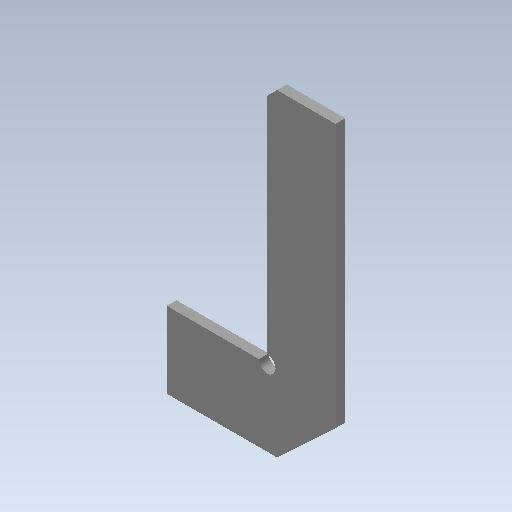
# Autodesk Inventor part: ADSK-MH-10038
Saved by Autodesk Inventor 2020.2 (Build 242310000, 310)
## iProperties
Created: 2008-03-27
Part Number: ADSK-MH-10038
Document SubType Name: Modeling
Designer: R.O'mahony
Density: 7.86 g/cm^3
Mass: 284.494 g
Surface Area: 169.314 cm^2
Volume: 36.1952 cm^3
Material: Steel, Mild
Appearance: Steel
Description: Back Transfer Support
Engineer: Demir Ali
Checked By: Demir Ali
Company: Autodesk Ltd
Author: R.O'mahony
Keywords: Roller Conveyor
Revision Number: A
Autodesk Inventor part; units mm, degrees
ref_plane "YZ Plane" through (0, 0, 0) normal (1, 0, 0) x (0, 1, 0)
ref_plane "XZ Plane" through (0, 0, 0) normal (0, 1, 0) x (-1, 0, 0)
ref_plane "XY Plane" through (0, 0, 0) normal (0, 0, 1) x (1, 0, 0)
sketch "Sketch1" plane through (0, 0, 0) normal (0, 0, 1) x (1, 0, 0)
  line L0 (2519.2496, -500.1029) -> (2519.2496, -385.3529)
  line L1 (2554.2496, -380.3529) -> (2524.2496, -380.3529)
  line L2 (2554.2496, -380.3529) -> (2554.2496, -515.3529)
  line L3 (2467.7344, -543.3529) -> (2524.2496, -543.3529)
  line L4 (2554.2496, -515.3529) -> (2524.2496, -543.3529)
  line L5 (2514.9996, -504.3529) -> (2467.7344, -504.3529)
  line L6 (2467.7344, -543.3529) -> (2467.7344, -504.3529)
  line L7 (2521.7496, -380.3529) -> (2519.2496, -384.3529)
  arc A0 (2514.9996, -504.3529) -> (2519.2496, -500.1029) centre (2519.2496, -504.3529) ccw
  line L8 (2519.2496, -385.3529) -> (2524.2496, -380.3529)
  point P0 (0, 0)
  point P1 (2519.2496, -380.3529)
  dimension "d1" = 35
  dimension "d3" = 135
  dimension "d5" = 163
  dimension "d7" = 51.5152
  dimension "d9" = 39
  dimension "d11" = 56.5152
  dimension "d13" = 8.5
  dimension "d16" = 5
  dimension "d17" = 5
  constraints: 18 end point, 4 point on line, 2 point on circle, 1 centre point, 1 perpendicular
  measures "d1" horizontal distance of L1.start L7.end
  measures "d3" distance of L1.start L2.end
  measures "d5" vertical distance of L1.start L3.end
  measures "d7" horizontal distance of L5.end L7.end
  measures "d9" distance of L5.end L3.start
  measures "d11" distance of L3.start L3.end
  measures "d13" diameter of A0
  measures "d16" distance of L0.end point (2519.25, -380.353)
  measures "d17" distance of L1.end point (2519.25, -380.353)
extrude "Extrusion1" add sketch "Sketch1" along normal blind 5
equation "\"d17\" = d16"
body "Solid1"
